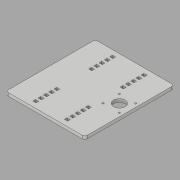
# Autodesk Inventor part: e_bot 1
Saved by Autodesk Inventor 2019 (Build 230136000, 136)
## iProperties
Created: 2021-11-03
Part Number: e_bot 1
Material: Generic
Document SubType Name: Modeling
Designer: Mohamed
Density: 1 g/cm^3
Appearance: Default
Author: Mohamed
Autodesk Inventor part; units mm, degrees
ref_plane "YZ Plane" through (0, 0, 0) normal (1, 0, 0) x (0, 1, 0)
ref_plane "XZ Plane" through (0, 0, 0) normal (0, 1, 0) x (-1, 0, 0)
ref_plane "XY Plane" through (0, 0, 0) normal (0, 0, 1) x (1, 0, 0)
sketch "Sketch1" plane through (0, 0, 0) normal (0, 1, 0) x (-1, 0, 0)
  line L0 (5, 0) -> (145, 0)
  line L1 (150, -5) -> (150, -145)
  line L2 (145, -150) -> (5, -150)
  line L3 (0, -145) -> (0, -5)
  arc A0 (150, -5) -> (145, 0) centre (145, -5) ccw
  arc A1 (145, -150) -> (150, -145) centre (145, -145) ccw
  arc A2 (5, 0) -> (0, -5) centre (5, -5) ccw
  arc A3 (0, -145) -> (5, -150) centre (5, -145) ccw
  circle A4 centre (128.033, -128.033) radius 5
  circle A5 centre (128.033, -21.967) radius 5
  circle A6 centre (21.967, -21.967) radius 5
  circle A7 centre (21.967, -128.033) radius 5
  point P0 (0, 0)
  point P1 (150, -150)
  point P2 (150, 0)
  point P3 (0, -150)
  dimension "d0" = 150
  dimension "d1" = 150
  dimension "d2" = 5
  dimension "d9" = 10
  dimension "d10" = 10
  dimension "d11" = 10
  dimension "d12" = 10
  constraints: 8 centre point, 8 end point, 8 point on circle, 8 point on line, 8 tangent, 3 equal radius, 2 parallel, 1 horizontal, 1 perpendicular
  measures "d0" distance of point (150, -150) point (0, -150)
  measures "d1" distance of point (150, 0) point (150, -150)
  measures "d2" radius of A0
  measures "d9" diameter of A4
  measures "d10" diameter of A5
  measures "d11" diameter of A6
  measures "d12" diameter of A7
extrude "Extrusion1" add sketch "Sketch1" along normal blind 6
sketch "Sketch2" plane through (0, 6, 0) normal (0, 1, 0) x (1, 0, 0)
  line L0 (0, 5) -> (0, 145) projected
  circle A0 centre (-21.967, 21.967) radius 5 projected
  circle A1 centre (-21.967, 77.828) radius 11
  circle A2 centre (-37.467, 62.328) radius 1.6
  circle A3 centre (-37.467, 93.328) radius 1.6
  circle A4 centre (-6.467, 62.328) radius 1.6
  circle A5 centre (-6.467, 93.328) radius 1.6
  point P0 (0, 0)
  dimension "d15" = 22
  dimension "d21" = 3.2
  dimension "d22" = 3.2
  dimension "d23" = 3.2
  dimension "d24" = 3.2
  constraints: 5 centre point
  measures "d15" diameter of A1
  measures "d21" diameter of A2
  measures "d22" diameter of A3
  measures "d23" diameter of A4
  measures "d24" diameter of A5
extrude "Extrusion2" cut sketch "Sketch2" against normal blind 6 contours A1 | A2 | A3 | A4 | A5
sketch "Sketch3" plane through (0, 6, 0) normal (0, 1, 0) x (1, 0, 0)
  circle A0 centre (-128.033, 128.033) radius 5 projected
  arc A1 (-145, 150) -> (-150, 145) centre (-145, 145) ccw projected
  line L0 (-150, 145) -> (0, 145)
  line L1 (0, 145) -> (0, 155)
  line L2 (-5, 160) -> (-145, 160)
  line L3 (-150, 155) -> (-150, 145)
  arc A2 (-150, 5) -> (-145, 0) centre (-145, 5) ccw projected
  line L4 (-150, 5) -> (0, 5)
  line L5 (0, 5) -> (0, -5)
  line L6 (-5, -10) -> (-145, -10)
  line L7 (-150, -5) -> (-150, 5)
  arc A3 (-145, 160) -> (-150, 155) centre (-145, 155) ccw
  arc A4 (0, 155) -> (-5, 160) centre (-5, 155) ccw
  arc A5 (-150, -5) -> (-145, -10) centre (-145, -5) ccw
  arc A6 (-5, -10) -> (0, -5) centre (-5, -5) ccw
  point P0 (0, 0)
  point P1 (0, 160)
  point P2 (-150, 160)
  point P3 (0, -10)
  point P4 (-150, -10)
  dimension "d29" = 150
  dimension "d30" = 15
  dimension "d31" = 150
  dimension "d32" = 15
  dimension "d33" = 5
  constraints: 16 end point, 8 point on circle, 8 point on line, 8 tangent, 4 centre point, 4 parallel, 3 equal radius, 2 horizontal, 2 perpendicular
  measures "d29" distance of point (-150, 160) point (0, 160)
  measures "d30" distance of point (0, 160) L0.end
  measures "d31" distance of point (0, -10) point (-150, -10)
  measures "d32" distance of L4.end point (0, -10)
  measures "d33" radius of A3
extrude "Extrusion3" add sketch "Sketch3" against normal blind 6 contours L3 A3 L2 A4 L1 L0 | L4 L5 A6 L6 A5 L7
sketch "Sketch4" plane through (0, 6, 0) normal (0, 1, 0) x (1, 0, 0)
  circle A0 centre (-128.033, 128.033) radius 5 projected
  line L0 (-108.033, 105.533) -> (-102.033, 105.533)
  line L1 (-102.033, 105.533) -> (-102.033, 110.533)
  line L2 (-102.033, 110.533) -> (-108.033, 110.533)
  line L3 (-108.033, 110.533) -> (-108.033, 105.533)
  circle A1 centre (-21.967, 128.033) radius 5 projected
  line L4 (-41.967, 105.533) -> (-47.967, 105.533)
  line L5 (-47.967, 105.533) -> (-47.967, 110.533)
  line L6 (-47.967, 110.533) -> (-41.967, 110.533)
  line L7 (-41.967, 110.533) -> (-41.967, 105.533)
  circle A2 centre (-128.033, 21.967) radius 5 projected
  line L8 (-108.033, -0.533) -> (-102.033, -0.533)
  line L9 (-102.033, -0.533) -> (-102.033, 4.467)
  line L10 (-102.033, 4.467) -> (-108.033, 4.467)
  line L11 (-108.033, 4.467) -> (-108.033, -0.533)
  circle A3 centre (-21.967, 21.967) radius 5 projected
  line L12 (-41.967, -0.533) -> (-47.967, -0.533)
  line L13 (-47.967, -0.533) -> (-47.967, 4.467)
  line L14 (-47.967, 4.467) -> (-41.967, 4.467)
  line L15 (-41.967, 4.467) -> (-41.967, -0.533)
  point P0 (0, 0)
  dimension "d39" = 6
  dimension "d40" = 5
  dimension "d43" = 6
  dimension "d44" = 5
  dimension "d47" = 6
  dimension "d48" = 5
  dimension "d51" = 6
  dimension "d52" = 5
  constraints: 32 end point, 8 parallel, 4 horizontal, 4 perpendicular
  measures "d39" distance of L2.end L1.end
  measures "d40" distance of L1.end L0.end
  measures "d43" distance of L5.end L6.end
  measures "d44" distance of L4.end L5.end
  measures "d47" distance of L10.end L9.end
  measures "d48" distance of L9.end L8.end
  measures "d51" distance of L13.end L14.end
  measures "d52" distance of L12.end L13.end
extrude "Extrusion4" cut sketch "Sketch4" against normal blind 6 contours L3 L2 L1 L0 | L4 L5 L6 L7 | L11 L10 L9 L8 | L12 L13 L14 L15
pattern_linear "Rectangular Pattern1" count 5 spacing 10 along (0, 0, -1) of "Extrusion4"
sketch "Sketch5" plane through (0, 6, 0) normal (0, 1, 0) x (1, 0, 0)
  circle A0 centre (-128.033, 21.967) radius 5 projected
  circle A1 centre (-128.033, 21.967) radius 5
  circle A2 centre (-128.033, 128.033) radius 5 projected
  circle A3 centre (-128.033, 128.033) radius 5
  circle A4 centre (-21.967, 128.033) radius 5 projected
  circle A5 centre (-21.967, 128.033) radius 5
  circle A6 centre (-21.967, 21.967) radius 5 projected
  circle A7 centre (-21.967, 21.967) radius 5
  point P0 (0, 0)
  dimension "d58" = 10
  dimension "d59" = 10
  dimension "d60" = 10
  dimension "d61" = 10
  constraints: 4 centre point, 4 coincident
  measures "d58" diameter of A1
  measures "d59" diameter of A3
  measures "d60" diameter of A5
  measures "d61" diameter of A7
extrude "Extrusion5" add sketch "Sketch5" against normal blind 6
body "Solid1"
